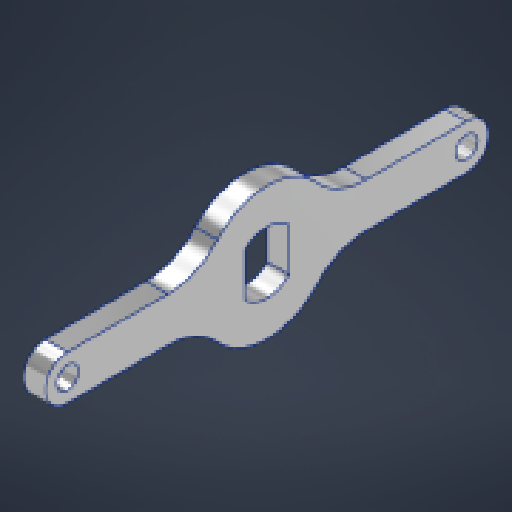
# Autodesk Inventor part: panel
Saved by Autodesk Inventor 2024 (Build 280153000, 153)
## iProperties
Created: 2024-05-05
Part Number: panel
Material: Aluminum 6061
Document SubType Name: Modeling
Designer: markm
Density: 2.7 g/cm^3
Appearance: Aluminum - Flat
Author: markm
Autodesk Inventor part; units mm, degrees
ref_plane "YZ Plane" through (0, 0, 0) normal (1, 0, 0) x (0, 1, 0)
ref_plane "XZ Plane" through (0, 0, 0) normal (0, 1, 0) x (-1, 0, 0)
ref_plane "XY Plane" through (0, 0, 0) normal (0, 0, 1) x (1, 0, 0)
sketch "Sketch4" plane through (0, 0, 0) normal (1, 0, 0) x (0, 1, 0)
  circle A0 centre (0, 0) radius 7
  line L0 (4.899, 5) -> (-4.899, 5)
  line L1 (-4.899, -5) -> (4.899, -5)
  circle A1 centre (0, 0) radius 15
  circle A2 centre (0, 45) radius 2.5
  circle A3 centre (0, 45) radius 5
  line L2 (5, 45) -> (5, 22.3607)
  line L3 (-5, 45) -> (-5, 22.3607)
  line L4 (0, 0) -> (0, 45) construction
  arc A4 (5, 22.3607) -> (10, 11.1803) centre (20, 22.3607) ccw
  arc A5 (-10, 11.1803) -> (-5, 22.3607) centre (-20, 22.3607) ccw
  dimension "d29" = 30
  dimension "d18" = 14
  dimension "d19" = 10
  dimension "d30" = 10
  dimension "d31" = 5
  dimension "d33" = 45
  constraints: 10 end point, 10 point on circle, 5 centre point, 3 coincident, 3 symmetric about line, 2 parallel, 2 tangent, 2 vertical, 1 horizontal, 7 other
  measures "d18" diameter of A0
  measures "d19" distance between parallel lines of L1 L0
  measures "d30" diameter of A3
  measures "d31" diameter of A2
  measures "d33" distance of L4.start L4.end
extrude "Extrusion4" add sketch "Sketch4" along normal mid plane 5 contours L0 A0 | A0 L1 | A1
extrude "Extrusion5" add sketch "Sketch4" along normal mid plane 5 contours A1 A5 L3 A3 L2 A4 | A3
mirror "Mirror2" about plane through (0, 0, 0) normal (0, 0, 1) of "Extrusion5"
body "Solid2"
